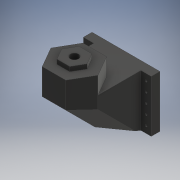
# Autodesk Inventor part: BA30
Saved by Autodesk Inventor 2017 (Build 210142000, 142)
## iProperties
Created: 2019-11-14
Part Number: BA30
Material: ABS Plastic
Document SubType Name: Modeling
Designer: Dell
Density: 1.06 g/cm^3
Appearance: Smooth - Black
Author: Dell
Autodesk Inventor part; units mm, degrees
ref_plane "YZ Plane" through (0, 0, 0) normal (1, 0, 0) x (0, 1, 0)
ref_plane "XZ Plane" through (0, 0, 0) normal (0, 1, 0) x (-1, 0, 0)
ref_plane "XY Plane" through (0, 0, 0) normal (0, 0, 1) x (1, 0, 0)
sketch "Sketch1" plane through (0, 0, 0) normal (0, 0, 1) x (1, 0, 0)
  line L0 (-36.9504, 0) -> (-18.4752, 32)
  line L1 (-18.4752, 32) -> (18.4752, 32)
  line L2 (18.4752, 32) -> (36.9504, 0)
  line L3 (36.9504, 0) -> (18.4752, -32)
  line L4 (18.4752, -32) -> (-18.4752, -32)
  line L5 (-18.4752, -32) -> (-36.9504, 0)
  circle A0 centre (0, 0) radius 12
  dimension "d0" = 64
  dimension "d1" = 24
  constraints: 12 end point, 2 coincident, 1 centre point, 1 horizontal, 13 other
  measures "d0" distance between parallel lines of L4 L1
  measures "d1" diameter of A0
extrude "Extrusion1" add sketch "Sketch1" along normal blind 13
sketch "Sketch2" plane through (0, 0, 0) normal (0, 0, -1) x (-1, 0, 0)
  line L0 (68.1273, 0) -> (34.0637, -59)
  line L1 (34.0637, -59) -> (-34.0637, -59)
  line L2 (-34.0637, -59) -> (-68.1273, 0)
  line L3 (-68.1273, 0) -> (-34.0637, 59)
  line L4 (-34.0637, 59) -> (34.0637, 59)
  line L5 (34.0637, 59) -> (68.1273, 0)
  circle A0 centre (0, 0) radius 12 projected
  line L6 (68.1273, 0) -> (68.1273, 149)
  line L7 (68.1273, 149) -> (-68.1273, 149)
  line L8 (-68.1273, 149) -> (-68.1273, 0)
  dimension "d4" = 118
  dimension "d8" = 90
  constraints: 18 end point, 2 perpendicular, 1 coincident, 1 horizontal, 1 vertical, 13 other
  measures "d4" distance between parallel lines of L4 L1
  measures "d8" distance between parallel lines of L7 L4
extrude "Extrusion2" add sketch "Sketch2" along normal blind 200
sketch "Sketch3" plane through (0, 0, -200) normal (0, 0, -1) x (-1, 0, 0)
  circle A0 centre (0, 0) radius 12 projected
extrude "Extrusion3" add sketch "Sketch3" against normal blind 120
sketch "Sketch4" plane through (0, 0, 0) normal (0, 0, 1) x (1, 0, 0)
  line L0 (68.1273, 0) -> (34.0637, -59)
  line L1 (34.0637, -59) -> (-34.0637, -59) construction
  line L2 (-34.0637, -59) -> (-68.1273, 0)
  line L3 (-68.1273, 0) -> (-34.0637, 59)
  line L4 (-34.0637, 59) -> (34.0637, 59)
  line L5 (34.0637, 59) -> (68.1273, 0)
  line L6 (68.1273, 0) -> (34.0637, -59) projected
  line L7 (68.1273, 149) -> (68.1273, 0) projected
  line L8 (68.1273, 0) -> (68.1273, 149)
  line L9 (-68.1273, 149) -> (68.1273, 149) projected
  line L10 (68.1273, 149) -> (-68.1273, 149)
  line L11 (-68.1273, 149) -> (-68.1273, 0)
  point P0 (0, 0)
  point P1 (0, 0)
  constraints: 18 end point, 2 coincident, 1 horizontal, 1 perpendicular, 1 vertical, 13 other
extrude "Extrusion4" cut sketch "Sketch4" against normal blind 50
chamfer "Chamfer1" distance 125 angle 45 1 edges at (0, -59, -200)
chamfer "Chamfer2" distance 34 angle 45 2 edges at (-68.1273, 33, -167) (68.1273, 33, -167)
sketch "Sketch5" plane through (-68.1273, 149, -200) normal (0, 1, 0) x (1, 0, 0)
  line L0 (0, -150) -> (0, 0) projected
  line L1 (0, 0) -> (-30, 0)
  line L2 (-30, 0) -> (-30, -150)
  line L3 (-30, -150) -> (0, -150)
  line L4 (0, -150) -> (0, 0)
  line L5 (0, 0) -> (136.2547, 0) projected
  line L6 (136.2547, 0) -> (166.2547, 0)
  line L7 (166.2547, 0) -> (166.2547, -150)
  line L8 (166.2547, -150) -> (136.2547, -150)
  line L9 (136.2547, -150) -> (136.2547, 0)
  circle A0 centre (151.2547, -131) radius 3
  circle A1 centre (151.2547, -103) radius 3
  circle A2 centre (151.2547, -75) radius 3
  circle A3 centre (151.2547, -47) radius 3
  circle A4 centre (151.2547, -19) radius 3
  line L10 (68.1273, -200) -> (68.1273, -239.5833)
  line L11 (0, 0) -> (-30, 0)
  line L12 (-30, 0) -> (-30, -150)
  line L13 (-30, -150) -> (0, -150)
  line L14 (0, -150) -> (0, 0)
  circle A5 centre (-15, -131) radius 3
  circle A6 centre (-15, -103) radius 3
  circle A7 centre (-15, -75) radius 3
  circle A8 centre (-15, -47) radius 3
  circle A9 centre (-15, -19) radius 3
  point P0 (151.2547, -150)
  point P1 (0, -150)
  point P2 (-15, -150)
  dimension "d19" = 30
  dimension "d20" = 30
  dimension "d21" = 6
  dimension "d22" = 19
  dimension "d25" = 28
  constraints: 26 end point, 10 centre point, 7 symmetric about line, 4 parallel, 2 coincident, 2 horizontal, 2 perpendicular, 2 vertical, 1 midpoint, 1 vertical alignment, 13 other
  measures "d19" distance of L2.end L0.start
  measures "d20" distance of L7.end L8.end
  measures "d21" diameter of A0
  measures "d22" distance from line of L8 A0.centre
  measures "d25" distance of A0.centre A1.centre
extrude "Extrusion5" add sketch "Sketch5" against normal blind 25
chamfer "Chamfer3" distance 58 angle 45 1 edges at (0, 66, -200)
body "Solid1"
